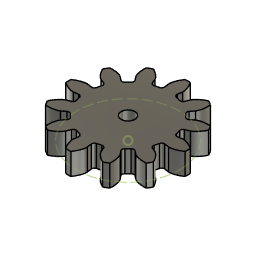
Axle gear (Autodesk Fusion 360 design; units mm, degrees)
description: Spur Gear; Module: 5.0; Num Teeth: 12; Pressure Angle: 20.0; Backlash: 0.00 mm
Autodesk Fusion 360 part; units mm, degrees
sketch "Sketch1" plane through (0, 0, 0) normal (0, 0, 1) x (1, 0, 0) in component "Spur Gear (12 teeth)"
  circle A0 centre (0, 0) radius 23.9492
  circle A1 centre (0, 0) radius 4
extrude "Extrude1" add sketch "Sketch1" along normal blind 12.7 in component "Spur Gear (12 teeth)"
sketch "Sketch2" plane through (0, 0, 0) normal (0, 0, 1) x (1, 0, 0) in component "Spur Gear (12 teeth)"
  spline S0 degree 5 poles (27.8917, -4.0958) (27.9119, -4.0987) (27.9524, -4.104) (28.0132, -4.11) (28.0947, -4.1142) (28.1969, -4.1144) (28.2993, -4.111) (28.402, -4.1054) (28.5047, -4.0986) (28.6075, -4.091) (28.7104, -4.0825) (28.8133, -4.0727) (28.9163, -4.0614) (29.0193, -4.0483) (29.1224, -4.0334) (29.2255, -4.0168) (29.3286, -3.9989) (29.4318, -3.9798) (29.5349, -3.9596) (29.638, -3.9385) (29.7411, -3.9163) (29.8441, -3.8931) (29.9472, -3.8688) (30.0502, -3.8434) (30.1531, -3.8168) (30.256, -3.7891) (30.3589, -3.7605) (30.4617, -3.7309) (30.5644, -3.7003) (30.667, -3.6688) (30.7696, -3.6365) (30.8721, -3.6032) (30.9746, -3.5689) (31.0769, -3.5338) (31.1792, -3.4978) (31.2813, -3.4608) (31.3834, -3.4231) (31.4854, -3.3844) (31.5872, -3.345) (31.689, -3.3047) (31.7906, -3.2635) (31.8922, -3.2216) (31.9936, -3.1788) (32.0949, -3.1353) (32.196, -3.0909) (32.2971, -3.0458) (32.398, -2.9999) (32.4987, -2.9532) (32.5994, -2.9057) (32.6999, -2.8575) (32.8002, -2.8086) (32.9004, -2.7589) (33.0005, -2.7084) (33.1003, -2.6572) (33.2001, -2.6053) (33.2997, -2.5527) (33.3991, -2.4993) (33.4983, -2.4452) (33.5974, -2.3905) (33.6964, -2.335) (33.7951, -2.2788) (33.8937, -2.2219) (33.9921, -2.1644) (34.0903, -2.1061) (34.1883, -2.0472) (34.2862, -1.9876) (34.3838, -1.9274) (34.4813, -1.8664) (34.5785, -1.8048) (34.6756, -1.7426) (34.7725, -1.6797) (34.8498, -1.6288) (34.9077, -1.5904) (34.9463, -1.5646) (34.9656, -1.5517) knots 0 0 0 0 0 0 0.01428571 0.02857143 0.04285714 0.05714286 0.07142857 0.08571429 0.1 0.11428571 0.12857143 0.14285714 0.15714286 0.17142857 0.18571429 0.2 0.21428571 0.22857143 0.24285714 0.25714286 0.27142857 0.28571429 0.3 0.31428571 0.32857143 0.34285714 0.35714286 0.37142857 0.38571429 0.4 0.41428571 0.42857143 0.44285714 0.45714286 0.47142857 0.48571429 0.5 0.51428571 0.52857143 0.54285714 0.55714286 0.57142857 0.58571429 0.6 0.61428571 0.62857143 0.64285714 0.65714286 0.67142857 0.68571429 0.7 0.71428571 0.72857143 0.74285714 0.75714286 0.77142857 0.78571429 0.8 0.81428571 0.82857143 0.84285714 0.85714286 0.87142857 0.88571429 0.9 0.91428571 0.92857143 0.94285714 0.95714286 0.97142857 0.98571429 1 1 1 1 1 1
  spline S1 degree 5 poles (27.8917, 4.0958) (27.9119, 4.0987) (27.9524, 4.104) (28.0132, 4.11) (28.0947, 4.1142) (28.1969, 4.1144) (28.2993, 4.111) (28.402, 4.1054) (28.5047, 4.0986) (28.6075, 4.091) (28.7104, 4.0825) (28.8133, 4.0727) (28.9163, 4.0614) (29.0193, 4.0483) (29.1224, 4.0334) (29.2255, 4.0168) (29.3286, 3.9989) (29.4318, 3.9798) (29.5349, 3.9596) (29.638, 3.9385) (29.7411, 3.9163) (29.8441, 3.8931) (29.9472, 3.8688) (30.0502, 3.8434) (30.1531, 3.8168) (30.256, 3.7891) (30.3589, 3.7605) (30.4617, 3.7309) (30.5644, 3.7003) (30.667, 3.6688) (30.7696, 3.6365) (30.8721, 3.6032) (30.9746, 3.5689) (31.0769, 3.5338) (31.1792, 3.4978) (31.2813, 3.4608) (31.3834, 3.4231) (31.4854, 3.3844) (31.5872, 3.345) (31.689, 3.3047) (31.7906, 3.2635) (31.8922, 3.2216) (31.9936, 3.1788) (32.0949, 3.1353) (32.196, 3.0909) (32.2971, 3.0458) (32.398, 2.9999) (32.4987, 2.9532) (32.5994, 2.9057) (32.6999, 2.8575) (32.8002, 2.8086) (32.9004, 2.7589) (33.0005, 2.7084) (33.1003, 2.6572) (33.2001, 2.6053) (33.2997, 2.5527) (33.3991, 2.4993) (33.4983, 2.4452) (33.5974, 2.3905) (33.6964, 2.335) (33.7951, 2.2788) (33.8937, 2.2219) (33.9921, 2.1644) (34.0903, 2.1061) (34.1883, 2.0472) (34.2862, 1.9876) (34.3838, 1.9274) (34.4813, 1.8664) (34.5785, 1.8048) (34.6756, 1.7426) (34.7725, 1.6797) (34.8498, 1.6288) (34.9077, 1.5904) (34.9463, 1.5646) (34.9656, 1.5517) knots 0 0 0 0 0 0 0.01428571 0.02857143 0.04285714 0.05714286 0.07142857 0.08571429 0.1 0.11428571 0.12857143 0.14285714 0.15714286 0.17142857 0.18571429 0.2 0.21428571 0.22857143 0.24285714 0.25714286 0.27142857 0.28571429 0.3 0.31428571 0.32857143 0.34285714 0.35714286 0.37142857 0.38571429 0.4 0.41428571 0.42857143 0.44285714 0.45714286 0.47142857 0.48571429 0.5 0.51428571 0.52857143 0.54285714 0.55714286 0.57142857 0.58571429 0.6 0.61428571 0.62857143 0.64285714 0.65714286 0.67142857 0.68571429 0.7 0.71428571 0.72857143 0.74285714 0.75714286 0.77142857 0.78571429 0.8 0.81428571 0.82857143 0.84285714 0.85714286 0.87142857 0.88571429 0.9 0.91428571 0.92857143 0.94285714 0.95714286 0.97142857 0.98571429 1 1 1 1 1 1
  arc A0 (34.9656, -1.5517) -> (34.9656, 1.5517) centre (0, 0) ccw
  line L0 (23.6852, -3.4795) -> (27.8917, -4.0958)
  line L1 (23.6852, 3.4795) -> (27.8917, 4.0958)
  line L2 (23.6852, -3.4795) -> (23.6852, 3.4795)
  point P0 (28.3816, -4.1063)
  point P1 (28.8788, -4.0653)
  point P2 (29.3803, -3.9892)
  point P3 (29.885, -3.8833)
  point P4 (30.3921, -3.7508)
  point P5 (30.9008, -3.5934)
  point P6 (31.4105, -3.4126)
  point P7 (31.9208, -3.2094)
  point P8 (32.4311, -2.9844)
  point P9 (32.9409, -2.7383)
  point P10 (33.4497, -2.4716)
  point P11 (33.957, -2.1848)
  point P12 (34.4625, -1.878)
  point P13 (28.3816, 4.1063)
  point P14 (28.8788, 4.0653)
  point P15 (29.3803, 3.9892)
  point P16 (29.885, 3.8833)
  point P17 (30.3921, 3.7508)
  point P18 (30.9008, 3.5934)
  point P19 (31.4105, 3.4126)
  point P20 (31.9208, 3.2094)
  point P21 (32.4311, 2.9844)
  point P22 (32.9409, 2.7383)
  point P23 (33.4497, 2.4716)
  point P24 (33.957, 2.1848)
  point P25 (34.4625, 1.878)
extrude "Extrude2" add sketch "Sketch2" along normal blind 12.7 in component "Spur Gear (12 teeth)"
fillet "Fillet1" radius 1.5875 2 edges at (23.6949, -3.481, 6.35) (23.6949, 3.481, 6.35) in component "Spur Gear (12 teeth)"
pattern_circular "C-Pattern1" count 12 over 360 about axis through (0, 0, 0) along (0, 0, 1) of "Extrude2", "Fillet1" in component "Spur Gear (12 teeth)"
sketch "Sketch3" plane through (0, 0, 0) normal (0, 0, 1) x (1, 0, 0) in component "Spur Gear (12 teeth)"
  circle A0 centre (0, 0) radius 30 construction
component "Spur Gear (12 teeth)" placed x (1, 0, 0) y (0, 1, 0) z (0, 0, 1) at (0, 0, 0)
